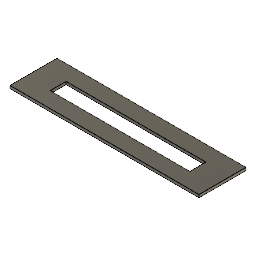
lan switch plate v1 (Autodesk Fusion 360 design; units mm, degrees)
Autodesk Fusion 360 part; units mm, degrees
sketch "Sketch1" plane through (0, 0, 0) normal (0, 0, 1) x (1, 0, 0)
  line L0 (0, 0) -> (609.6, 0)
  line L1 (609.6, 0) -> (609.6, 152.4)
  line L2 (609.6, 152.4) -> (0, 152.4)
  line L3 (0, 152.4) -> (0, 0)
  line L4 (0, 0) -> (0, 53.848)
  line L5 (0, 76.2) -> (609.6, 76.2) construction
  line L6 (304.8, 152.4) -> (304.8, 0) construction
  line L7 (529.8, 101.6) -> (79.8, 101.6)
  line L8 (79.8, 101.6) -> (79.8, 50.8)
  line L9 (79.8, 50.8) -> (529.8, 50.8)
  line L10 (529.8, 50.8) -> (529.8, 101.6)
  line L11 (529.8, 101.6) -> (79.8, 50.8) construction
  line L12 (79.8, 101.6) -> (529.8, 50.8) construction
  point P0 (0, 0)
  dimension "d1" = 609.6
  dimension "d2" = 152.4
  dimension "d12" = 450
  dimension "d13" = 50.8
  measures "d1" distance of P0
  measures "d12" distance of P0
extrude "Extrude1" add sketch "Sketch1" along normal blind 9.525
equation "d1 = 2'-0\""
equation "d2 = 6\""
equation "d8 = ( 3 / 8 ) * 1 in"
